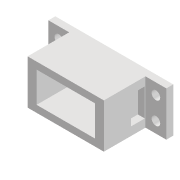
# Autodesk Inventor part: base
Saved by Autodesk Inventor 2022 (Build 260153000, 153)
## iProperties
Created: 2022-03-09
Part Number: base
Material: Generic
Document SubType Name: Modeling
Designer: piers
Density: 1 g/cm^3
Appearance: Default
Author: piers
Autodesk Inventor part; units mm, degrees
ref_plane "YZ Plane" through (0, 0, 0) normal (1, 0, 0) x (0, 1, 0)
ref_plane "XZ Plane" through (0, 0, 0) normal (0, 1, 0) x (-1, 0, 0)
ref_plane "XY Plane" through (0, 0, 0) normal (0, 0, 1) x (1, 0, 0)
sketch "Sketch1" plane through (0, 0, 0) normal (0, 0, 1) x (1, 0, 0)
  line L0 (0, 0) -> (42, 0)
  line L1 (42, 0) -> (42, 22)
  line L2 (42, 22) -> (0, 22)
  line L3 (0, 22) -> (0, 0)
  line L4 (0, 0) -> (-6.5, 0)
  line L5 (-6.5, 0) -> (-6.5, 27)
  line L6 (-6.5, 27) -> (48.5, 27)
  line L7 (48.5, 27) -> (48.5, -5)
  line L8 (48.5, -5) -> (-6.5, -5)
  line L9 (-6.5, -5) -> (-6.5, 0)
  line L10 (-6.5, 27) -> (-21.5, 27)
  line L11 (-21.5, 27) -> (-21.5, -5)
  line L12 (-21.5, -5) -> (-6.5, -5)
  line L13 (48.5, -5) -> (63.5, -5)
  line L14 (63.5, -5) -> (63.5, 27)
  line L15 (63.5, 27) -> (48.5, 27)
  circle A0 centre (-14, 19) radius 3.1
  circle A1 centre (-14, 3) radius 3.1
  line L16 (21, 22) -> (21, 19)
  circle A2 centre (56, 19) radius 3.1
  circle A3 centre (56, 3) radius 3.1
  dimension "d0" = 42
  dimension "d1" = 22
  dimension "d2" = 6.5
  dimension "d3" = 27
  dimension "d4" = 55
  dimension "d5" = 32
  dimension "d11" = 15
  dimension "d12" = 15
  dimension "d13" = 32
  dimension "d16" = 7.5
  dimension "d17" = 7.5
  dimension "d18" = 8
  dimension "d19" = 8
  dimension "d20" = 6.2
  dimension "d21" = 6.2
  constraints: 34 end point, 5 parallel, 5 perpendicular, 4 centre point, 4 horizontal, 2 symmetric about line, 1 midpoint, 1 point on line, 1 vertical, 2 other
  measures "d0" distance of L2.end L1.end
  measures "d1" distance of L0.end L1.end
  measures "d2" distance of L0.start L4.end
  measures "d3" distance of L4.end L5.end
  measures "d4" distance of L5.end L6.end
  measures "d5" distance of L6.end L7.end
  measures "d11" distance of L5.end L10.end
  measures "d12" distance of L7.end L13.end
  measures "d13" distance of L13.end L14.end
  measures "d16" distance from line of A1.centre L5
  measures "d17" distance from line of A0.centre L5
  measures "d18" distance from line of L10 A0.centre
  measures "d19" distance from line of L12 A1.centre
  measures "d20" diameter of A0
  measures "d21" diameter of A1
extrude "Extrusion1" add sketch "Sketch1" along normal blind 30 contours L5 L6 L7 L8 L9
extrude "Extrusion2" add sketch "Sketch1" against normal blind 5 contours L3 L2 L1 L0 | L5 L6 L7 L8 L9
extrude "Extrusion3" add sketch "Sketch1" against normal blind 5 contours L9 L12 L11 L10 L5 | L15 L14 L13 L7
sketch "Sketch2" plane through (48.5, -5, 30) normal (1, 0, 0) x (0, 0, -1)
  line L0 (29.5, 26) -> (19.5, 26) projected
  line L1 (19.5, 26) -> (19.5, 6) projected
  line L2 (19.5, 6) -> (29.5, 6) projected
  line L3 (29.5, 6) -> (29.5, 26) projected
  point P0 (30, 5)
extrude "Extrusion4" cut sketch "Sketch2" against normal blind 5
equation "\"d2\" = -0.5 * d0 + 0.5 * d4"
equation "\"d21\" = d20"
body "Solid1"
